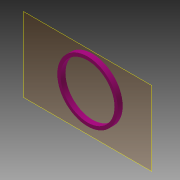
# Autodesk Inventor part: Big Bearing Spacer
Saved by Autodesk Inventor 2014 (Build 180170000, 170)
## iProperties
Created: 2015-02-14
Part Number: Big Bearing Spacer
Material: Generic
Document SubType Name: Modeling
Designer: Spooner
Density: 1 g/cm^3
Appearance: Magenta
Author: Spooner
Autodesk Inventor part; units mm, degrees
ref_plane "YZ Plane" through (0, 0, 0) normal (1, 0, 0) x (0, 1, 0)
ref_plane "XZ Plane" through (0, 0, 0) normal (0, 1, 0) x (-1, 0, 0)
ref_plane "XY Plane" through (0, 0, 0) normal (0, 0, 1) x (1, 0, 0)
ref_plane "Work Plane1" through (0, 0, 0) normal (0, 0, 1) x (1, 0, 0)
sketch "Sketch1" plane through (0, 0, 0) normal (0, 0, 1) x (1, 0, 0)
  circle A0 centre (0, 0) radius 23.495 projected
  circle A1 centre (-36.957, 0) radius 4.191 projected
  circle A2 centre (36.957, 0) radius 4.191 projected
  arc A3 (45.339, 6.35) -> (42.164, 9.525) centre (42.164, 6.35) ccw projected
  line L0 (42.164, 9.525) -> (38.1051, 9.525) projected
  arc A4 (19.3802, 17.7628) -> (38.1051, 9.525) centre (38.1051, 34.925) ccw projected
  arc A5 (19.3802, 17.7628) -> (-19.3802, 17.7628) centre (0, 0) ccw projected
  arc A6 (-38.1051, 9.525) -> (-19.3802, 17.7628) centre (-38.1051, 34.925) ccw projected
  line L1 (-38.1051, 9.525) -> (-42.164, 9.525) projected
  arc A7 (-42.164, 9.525) -> (-45.339, 6.35) centre (-42.164, 6.35) ccw projected
  line L2 (-45.339, 6.35) -> (-45.339, -6.35) projected
  arc A8 (-45.339, -6.35) -> (-42.164, -9.525) centre (-42.164, -6.35) ccw projected
  line L3 (-42.164, -9.525) -> (-38.1051, -9.525) projected
  arc A9 (-19.3802, -17.7628) -> (-38.1051, -9.525) centre (-38.1051, -34.925) ccw projected
  arc A10 (-19.3802, -17.7628) -> (19.3802, -17.7628) centre (0, 0) ccw projected
  arc A11 (38.1051, -9.525) -> (19.3802, -17.7628) centre (38.1051, -34.925) ccw projected
  line L4 (38.1051, -9.525) -> (42.164, -9.525) projected
  arc A12 (42.164, -9.525) -> (45.339, -6.35) centre (42.164, -6.35) ccw projected
  line L5 (45.339, -6.35) -> (45.339, 6.35) projected
  circle A13 centre (0, 0) radius 23.749 projected
  circle A14 centre (0, 0) radius 20.955
  point P0 (0, 0)
  dimension "d0" = 2.54
  constraints: 1 centre point, 1 coincident
  measures "d0" radial gap between concentric circles of A14 A0
extrude "Extrusion1" add sketch "Sketch1" against normal blind 3.81 contours A0
body "Solid1"
